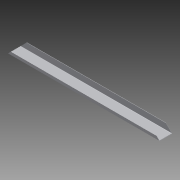
# Autodesk Inventor part: tableSide
Saved by Autodesk Inventor 2013 (Build 170138000, 138)
## iProperties
Created: 2012-10-20
Part Number: tableSide
Material: Aluminum 6061
Document SubType Name: Sheet Metal
Designer: Istvan
Density: 2.71 g/cm^3
Sheet Metal Rule: Default
Flat Pattern Width: 17.1904 cm
Flat Pattern Length: 121.92 cm
Flat Pattern Area: 2095.85 cm^2
Sheet Metal Width: 6.768 in
Sheet Metal Length: 48.000 in
Sheet Metal Area: 324.858 in^2
Author: Istvan
Autodesk Inventor part; units mm, degrees
ref_plane "YZ Plane" through (0, 0, 0) normal (1, 0, 0) x (0, 1, 0)
ref_plane "XZ Plane" through (0, 0, 0) normal (0, 1, 0) x (-1, 0, 0)
ref_plane "XY Plane" through (0, 0, 0) normal (0, 0, 1) x (1, 0, 0)
sketch "Sketch1" plane through (0, 0, 0) normal (0, 1, 0) x (-1, 0, 0)
  line L0 (0, 0) -> (1219.2, 0)
  line L1 (1219.2, 0) -> (1219.2, 101.6)
  line L2 (1219.2, 101.6) -> (0, 101.6)
  line L3 (0, 101.6) -> (0, 0)
  dimension "d0" = 1219.2
  dimension "d1" = 101.6
  measures "d0" distance of L2.end L1.end
  measures "d1" distance of L1.end L0.end
extrude "Plate1" add sketch "Sketch1" along normal blind 2.3813
sketch "Sketch2" plane through (-1219.2, 0, 2.3813) normal (0, 0, -1) x (-1, 0, 0)
  line L0 (-1219.2, 0) -> (0, 0)
  line L1 (0, 0) -> (0, 50.8)
  line L2 (0, 50.8) -> (-1219.2, 50.8)
  line L3 (-1219.2, 50.8) -> (-1219.2, 0)
  constraints: 6 end point, 1 horizontal, 1 perpendicular, 1 vertical
edge flange "Flange1" height 50.8 angle 90 thickness 2.3813 bend radius 2.3813 thickness toward (0, 0, -1) relief straight relief width 2.3813 relief depth 1.1906 edges at (-609.6, 2.3813, 0) wall of the first edge with corners at (0, 0, 2.3813) (-1219.2, 0, 2.3813) (-1219.2, 50.8, 2.3812) (0, 50.8, 2.3812)
bend "Bend1"
corner "Corner1"
sketch "Sketch3" plane through (0, 2.3813, 101.6) normal (0, 0, 1) x (1, 0, 0)
  line L0 (-1219.2, 0) -> (0, 0)
  line L1 (0, 0) -> (0, 23.0187)
  line L2 (0, 23.0187) -> (-1219.2, 23.0187)
  line L3 (-1219.2, 23.0187) -> (-1219.2, 0)
  constraints: 6 end point, 1 horizontal, 1 perpendicular, 1 vertical
edge flange "Flange2" height 25.4 angle 90 thickness 2.3813 bend radius 2.3813 thickness toward (0, 0, 1) relief straight relief width 2.3813 relief depth 1.1906 edges at (-609.6, 2.3813, 101.6) wall of the first edge with corners at (-1219.2, 2.3813, 101.6) (0, 2.3813, 101.6) (0, 25.4, 101.6) (-1219.2, 25.4, 101.6)
bend "Bend2"
corner "Corner2"
sketch "Sketch4" plane through (0, 50.8, 0) normal (0, 0, -1) x (-1, 0, 0)
  line L0 (0, 0) -> (1219.2, 0) projected
  line L1 (1219.2, -50.8) -> (0, -50.8) projected
  line L2 (1219.2, 0) -> (1219.2, -46.0375) projected
  line L3 (1219.2, -50.8) -> (1219.2, -46.0375) projected
  line L4 (0, -46.0375) -> (0, -50.8) projected
  line L5 (0, -46.0375) -> (0, 0) projected
  line L6 (0, -50.8) -> (50.8, 0)
  line L7 (1219.2, -50.8) -> (1168.4, 0)
  dimension "d24" = 45
  dimension "d25" = 45
  constraints: 4 end point, 2 point on line
  measures "d24" angle of L5 L6
  measures "d25" angle of L7 L2
extrude "Extrusion1" cut sketch "Sketch4" against normal through all contours L0 L6 L4 L5 | L0 L2 L3 L7
equation "\"d25\" = d24"
equation "\"d3\" = BendReliefWidth"
equation "\"d4\" = BendReliefDepth"
equation "\"d5\" = MinimumRemnant"
equation "\"d6\" = BendRadius"
equation "\"d9\" = BendRadius"
equation "\"d10\" = CornerReliefSize"
equation "\"d11\" = GapSize"
equation "\"d12\" = JacobiRadiusSize"
equation "\"d13\" = BendReliefWidth"
equation "\"d14\" = BendReliefDepth"
equation "\"d15\" = MinimumRemnant"
equation "\"d16\" = BendRadius"
equation "\"d19\" = BendRadius"
equation "\"d20\" = CornerReliefSize"
equation "\"d21\" = GapSize"
equation "\"d22\" = JacobiRadiusSize"
equation "\"BendRadius\" = Thickness"
equation "\"BendReliefWidth\" = Thickness"
equation "\"BendReliefDepth\" = 0.5 * Thickness"
equation "\"CornerReliefSize\" = 4 * Thickness"
equation "\"MinimumRemnant\" = 2 * Thickness"
equation "\"TransitionRadius\" = BendRadius"
equation "\"JacobiRadiusSize\" = BendRadius"
equation "\"GapSize\" = Thickness"
equation "\"d2\" = BendRadius"
equation "\"Thickness\" = 2.38125"
body "Solid1"
